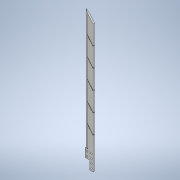
# Autodesk Inventor part: blade c 3.25
Saved by Autodesk Inventor 2021 (Build 250183000, 183)
## iProperties
Created: 2021-04-05
Part Number: blade c 3.25
Material: Generic
Document SubType Name: Modeling
Designer: newic
Density: 1 g/cm^3
Appearance: Default
Author: newic
Autodesk Inventor part; units mm, degrees
ref_plane "YZ Plane" through (0, 0, 0) normal (1, 0, 0) x (0, 1, 0)
ref_plane "XZ Plane" through (0, 0, 0) normal (0, 1, 0) x (-1, 0, 0)
ref_plane "XY Plane" through (0, 0, 0) normal (0, 0, 1) x (1, 0, 0)
sketch "Sketch1" plane through (0, 0, 0) normal (0, 0, 1) x (1, 0, 0)
  line L0 (0, 0) -> (88.9, 0)
  line L1 (88.9, 0) -> (88.9, 1168.4)
  line L2 (0, 1168.4) -> (0, 0)
  line L3 (-1378.8531, -765.1447) -> (-1378.8531, 1773.0142) construction
  line L4 (-1378.8531, 1773.0142) -> (415.5122, 1773.0142) construction
  line L5 (415.5122, 1773.0142) -> (415.5122, -765.1447) construction
  line L6 (415.5122, -765.1447) -> (-1378.8531, -765.1447) construction
  line L7 (44.45, 1168.4) -> (176.9474, 1168.4) construction
  line L8 (0, 1168.4) -> (0, 1119.7734)
  line L9 (88.9, 1168.4) -> (0, 1274.3469)
  line L10 (0, 1168.4) -> (0, 1274.3469)
  line L11 (88.9, 1168.4) -> (88.9, 1229.5585)
  line L12 (88.9, 1168.4) -> (88.9, 965.2)
  line L13 (88.9, 965.2) -> (88.9, 762)
  line L14 (88.9, 762) -> (88.9, 558.8)
  line L15 (88.9, 558.8) -> (88.9, 355.6)
  line L16 (88.9, 355.6) -> (88.9, 152.4)
  line L17 (88.9, 965.2) -> (-57.897, 1140.1458)
  line L18 (88.9, 965.2) -> (317.2756, 965.2) construction
  line L19 (88.9, 762) -> (-57.897, 936.9458)
  line L20 (88.9, 762) -> (317.2756, 762) construction
  line L21 (88.9, 558.8) -> (-71.0436, 749.4133)
  line L22 (88.9, 558.8) -> (337.728, 558.8) construction
  line L23 (88.9, 355.6) -> (-47.9591, 518.7023)
  line L24 (88.9, 355.6) -> (301.815, 355.6) construction
  line L25 (88.9, 152.4) -> (-31.1466, 295.4659)
  line L26 (88.9, 152.4) -> (275.6593, 152.4) construction
  line L27 (88.9, 152.4) -> (137.8508, 94.0627)
  line L28 (88.9, 355.6) -> (128.9332, 307.8903)
  line L29 (88.9, 558.8) -> (137.8508, 500.4627)
  line L30 (88.9, 762) -> (152.1538, 686.617)
  line L31 (-57.897, 936.9458) -> (152.1538, 686.617)
  line L32 (-71.0436, 749.4133) -> (137.8508, 500.4627)
  line L33 (-47.9591, 518.7023) -> (128.9332, 307.8903)
  line L34 (-31.1466, 295.4659) -> (137.8508, 94.0627)
  line L35 (164.9833, 874.5275) -> (-78.8863, 1165.1599)
  line L36 (90.3593, 966.4245) -> (-56.4377, 1141.3704)
  line L37 (87.4407, 963.9755) -> (-59.3563, 1138.9213)
  line L38 (157.3047, 680.4784) -> (-71.0436, 952.6133)
  line L39 (158.764, 681.7029) -> (-69.5842, 953.8378)
  line L40 (155.8454, 679.2539) -> (-72.5029, 951.3888)
  line L41 (144.9042, 492.0568) -> (-84.555, 765.5156)
  line L42 (146.3635, 493.2813) -> (-83.0956, 766.7401)
  line L43 (143.4449, 490.8323) -> (-86.0143, 764.2911)
  line L44 (137.8508, 297.2627) -> (-69.5842, 544.4742)
  line L45 (139.3101, 298.4872) -> (-68.1249, 545.6987)
  line L46 (136.3915, 296.0382) -> (-71.0436, 543.2497)
  line L47 (-41.5719, 307.8903) -> (172.2961, 53.0124)
  line L48 (-40.1126, 309.1148) -> (173.7555, 54.2369)
  line L49 (-43.0312, 306.6658) -> (170.8368, 51.7878)
  line L50 (87.4407, 963.9755) -> (94.264, 955.8438)
  dimension "d0" = 88.9
  dimension "d1" = 1168.4
  dimension "d23" = 40
  dimension "d37" = 1.905
  dimension "d38" = 1.905
  dimension "d39" = 1.905
  dimension "d40" = 1.905
  dimension "d41" = 1.905
  dimension "d42" = 1.905
  dimension "d43" = 1.905
  dimension "d44" = 1.905
  dimension "d45" = 1.905
  dimension "d46" = 1.905
  constraints: 94 end point, 11 parallel, 9 point on line, 7 horizontal, 5 equal length, 4 collinear, 3 vertical, 1 perpendicular, 2 other
  measures "d0" distance of L2.start L1.end
  measures "d1" distance of L1.end L0.end
  measures "d23" angle of L9 L11
  measures "d37" distance between parallel lines of L17 L36
  measures "d38" distance between parallel lines of L17 L37
  measures "d39" distance between parallel lines of L38 L39
  measures "d40" distance between parallel lines of L38 L40
  measures "d41" distance between parallel lines of L41 L42
  measures "d42" distance between parallel lines of L41 L43
  measures "d43" distance between parallel lines of L44 L45
  measures "d44" distance between parallel lines of L44 L46
  measures "d45" distance between parallel lines of L47 L48
  measures "d46" distance between parallel lines of L47 L49
extrude "Extrusion1" add sketch "Sketch1" along normal blind 15.875
sketch "Sketch2" plane through (0, 0, 15.875) normal (0, 0, 1) x (1, 0, 0)
  line L0 (0, 0) -> (88.9, 0)
  line L1 (88.9, 0) -> (88.9, 1168.4)
  line L2 (0, 1168.4) -> (0, 0)
  line L3 (-1378.8531, -765.1447) -> (-1378.8531, 1773.0142) construction
  line L4 (-1378.8531, 1773.0142) -> (415.5122, 1773.0142) construction
  line L5 (415.5122, 1773.0142) -> (415.5122, -765.1447) construction
  line L6 (415.5122, -765.1447) -> (-1378.8531, -765.1447) construction
  line L7 (44.45, 1168.4) -> (176.9474, 1168.4) construction
  line L8 (0, 1168.4) -> (0, 1119.7734)
  line L9 (88.9, 1168.4) -> (0, 1274.3469)
  line L10 (0, 1168.4) -> (0, 1274.3469)
  line L11 (88.9, 1168.4) -> (88.9, 1229.5585)
  line L12 (88.9, 1168.4) -> (88.9, 965.2)
  line L13 (88.9, 965.2) -> (88.9, 762)
  line L14 (88.9, 762) -> (88.9, 558.8)
  line L15 (88.9, 558.8) -> (88.9, 355.6)
  line L16 (88.9, 355.6) -> (88.9, 152.4)
  line L17 (88.9, 965.2) -> (-57.897, 1140.1458)
  line L18 (88.9, 965.2) -> (317.2756, 965.2) construction
  line L19 (88.9, 762) -> (-57.897, 936.9458)
  line L20 (88.9, 762) -> (317.2756, 762) construction
  line L21 (88.9, 558.8) -> (-71.0436, 749.4133)
  line L22 (88.9, 558.8) -> (337.728, 558.8) construction
  line L23 (88.9, 355.6) -> (-47.9591, 518.7023)
  line L24 (88.9, 355.6) -> (301.815, 355.6) construction
  line L25 (88.9, 152.4) -> (-31.1466, 295.4659)
  line L26 (88.9, 152.4) -> (275.6593, 152.4) construction
  line L27 (88.9, 152.4) -> (137.8508, 94.0627)
  line L28 (88.9, 355.6) -> (128.9332, 307.8903)
  line L29 (88.9, 558.8) -> (137.8508, 500.4627)
  line L30 (88.9, 762) -> (152.1538, 686.617)
  line L31 (-57.897, 936.9458) -> (152.1538, 686.617)
  line L32 (-71.0436, 749.4133) -> (137.8508, 500.4627)
  line L33 (-47.9591, 518.7023) -> (128.9332, 307.8903)
  line L34 (-31.1466, 295.4659) -> (137.8508, 94.0627)
  line L35 (164.9833, 874.5275) -> (-78.8863, 1165.1599)
  line L36 (90.3593, 966.4245) -> (-56.4377, 1141.3704)
  line L37 (87.4407, 963.9755) -> (-59.3563, 1138.9213)
  line L38 (157.3047, 680.4784) -> (-71.0436, 952.6133)
  line L39 (158.764, 681.7029) -> (-69.5842, 953.8378)
  line L40 (155.8454, 679.2539) -> (-72.5029, 951.3888)
  line L41 (144.9042, 492.0568) -> (-84.555, 765.5156)
  line L42 (146.3635, 493.2813) -> (-83.0956, 766.7401)
  line L43 (143.4449, 490.8323) -> (-86.0143, 764.2911)
  line L44 (137.8508, 297.2627) -> (-69.5842, 544.4742)
  line L45 (139.3101, 298.4872) -> (-68.1249, 545.6987)
  line L46 (136.3915, 296.0382) -> (-71.0436, 543.2497)
  line L47 (-41.5719, 307.8903) -> (172.2961, 53.0124)
  line L48 (-40.1126, 309.1148) -> (173.7555, 54.2369)
  line L49 (-43.0312, 306.6658) -> (170.8368, 51.7878)
  line L50 (87.4407, 963.9755) -> (94.264, 955.8438)
  point P0 (88.9, 962.2363)
  point P1 (88.9, 968.1637)
  point P2 (0, 1074.1105)
  point P3 (0, 1068.1832)
  point P4 (0, 864.9832)
  point P5 (88.9, 759.0363)
  point P6 (88.9, 764.9637)
  point P7 (0, 870.9105)
  point P8 (0, 661.7832)
  point P9 (88.9, 555.8363)
  point P10 (88.9, 561.7637)
  point P11 (0, 667.7105)
  point P12 (0, 458.5832)
  point P13 (88.9, 352.6363)
  point P14 (88.9, 358.5637)
  point P15 (0, 464.5105)
  point P16 (88.9, 155.3637)
  point P17 (0, 261.3105)
  point P18 (0, 255.3832)
  point P19 (88.9, 149.4363)
  dimension "d49" = 88.9
  dimension "d50" = 1168.4
  dimension "d51" = 40
  dimension "d52" = 1.905
  dimension "d53" = 1.905
  dimension "d54" = 1.905
  dimension "d55" = 1.905
  dimension "d56" = 1.905
  dimension "d57" = 1.905
  dimension "d58" = 1.905
  dimension "d59" = 1.905
  dimension "d60" = 1.905
  dimension "d61" = 1.905
  constraints: 94 end point, 11 parallel, 9 point on line, 7 horizontal, 5 equal length, 4 collinear, 3 vertical, 1 perpendicular, 2 other
  measures "d49" distance of L2.start L1.end
  measures "d50" distance of L1.end L0.end
  measures "d51" angle of L9 L11
  measures "d52" distance between parallel lines of L17 L36
  measures "d53" distance between parallel lines of L17 L37
  measures "d54" distance between parallel lines of L38 L39
  measures "d55" distance between parallel lines of L38 L40
  measures "d56" distance between parallel lines of L41 L42
  measures "d57" distance between parallel lines of L41 L43
  measures "d58" distance between parallel lines of L44 L45
  measures "d59" distance between parallel lines of L44 L46
  measures "d60" distance between parallel lines of L47 L48
  measures "d61" distance between parallel lines of L47 L49
extrude "Extrusion2" cut sketch "Sketch2" against normal blind 1.27 contours L2 L25 L1 L49 | L2 L48 L1 L25 | L2 L23 L1 L46 | L2 L45 L1 L23 | L2 L21 L1 L43 | L2 L42 L1 L21 | L2 L19 L1 L40 | L2 L39 L1 L19 | L2 L17 L1 L50 L37 | L2 L36 L1 L17
sketch "Sketch3" plane through (0, 0, 0) normal (0, 0, -1) x (-1, 0, 0)
  line L0 (-88.9, 149.4363) -> (0, 255.3832) projected
  line L1 (0, 261.3105) -> (-88.9, 155.3637) projected
  line L2 (0, 464.5105) -> (-88.9, 358.5637) projected
  line L3 (-88.9, 352.6363) -> (0, 458.5832) projected
  line L4 (-88.9, 555.8363) -> (0, 661.7832) projected
  line L5 (0, 667.7105) -> (-88.9, 561.7637) projected
  line L6 (-88.9, 759.0363) -> (0, 864.9832) projected
  line L7 (0, 870.9105) -> (-88.9, 764.9637) projected
  line L8 (-88.9, 962.2363) -> (0, 1068.1832) projected
  line L9 (0, 1074.1105) -> (-88.9, 968.1637) projected
  line L10 (0, 1274.3469) -> (0, 0) projected
  line L11 (-88.9, 1168.4) -> (0, 1274.3469) projected
  line L12 (-88.9, 0) -> (-88.9, 1168.4) projected
  line L13 (0, 0) -> (-88.9, 0) projected
extrude "Extrusion3" cut sketch "Sketch3" against normal blind 1.27 contours L12 L1 L10 L0 | L12 L2 L10 L3 | L12 L5 L10 L4 | L12 L7 L10 L6 | L12 L9 L10 L8
sketch "Sketch4" plane through (88.9, 968.1637, 15.875) normal (1, 0, 0) x (0, 0, -1)
  line L0 (-0.8567, 45.5077) -> (24.5433, 45.5077)
  line L1 (24.5433, 45.5077) -> (24.5433, 51.2227)
  line L2 (24.5433, 51.2227) -> (-0.8567, 51.2227)
  line L3 (-0.8567, 51.2227) -> (-0.8567, 45.5077)
  line L4 (1.27, -5.9273) -> (0, -5.9273) projected
  line L5 (0, -5.9273) -> (0, -4.4033)
  line L6 (0, 100.0196) -> (0, -97.2531) projected
  line L7 (-3.6064, -4.4033) -> (23.6569, -4.4033)
  line L8 (23.6569, -4.4033) -> (23.6569, 1.3117)
  line L9 (23.6569, 1.3117) -> (-3.6064, 1.3117)
  line L10 (-3.6064, 1.3117) -> (-3.6064, -4.4033)
  line L11 (1.27, -818.7273) -> (0, -818.7273) projected
  line L12 (0, -818.7273) -> (0, -817.2033)
  line L13 (0, -712.7804) -> (0, -968.1637) projected
  line L14 (1.27, -615.5273) -> (0, -615.5273) projected
  line L15 (0, -615.5273) -> (0, -614.0033)
  line L16 (0, -615.5273) -> (0, -509.5804) projected
  line L17 (1.27, -412.3273) -> (0, -412.3273) projected
  line L18 (0, -412.3273) -> (0, -410.8033)
  line L19 (0, -306.3804) -> (0, -503.6531) projected
  line L20 (1.27, -209.1273) -> (0, -209.1273) projected
  line L21 (0, -209.1273) -> (0, -207.6033)
  line L22 (0, -103.1804) -> (0, -300.4531) projected
  line L23 (-2.1765, -817.2033) -> (18.224, -817.2033)
  line L24 (18.224, -817.2033) -> (18.224, -811.4883)
  line L25 (18.224, -811.4883) -> (-2.1765, -811.4883)
  line L26 (-2.1765, -811.4883) -> (-2.1765, -817.2033)
  line L27 (-1.5796, -614.0033) -> (23.8204, -614.0033)
  line L28 (23.8204, -614.0033) -> (23.8204, -608.2883)
  line L29 (23.8204, -608.2883) -> (-1.5796, -608.2883)
  line L30 (-1.5796, -608.2883) -> (-1.5796, -614.0033)
  line L31 (-2.2774, -410.8033) -> (22.0155, -410.8033)
  line L32 (22.0155, -410.8033) -> (22.0155, -405.0883)
  line L33 (22.0155, -405.0883) -> (-2.2774, -405.0883)
  line L34 (-2.2774, -405.0883) -> (-2.2774, -410.8033)
  line L35 (-1.5796, -207.6033) -> (20.5708, -207.6033)
  line L36 (20.5708, -207.6033) -> (20.5708, -201.8883)
  line L37 (20.5708, -201.8883) -> (-1.5796, -201.8883)
  line L38 (-1.5796, -201.8883) -> (-1.5796, -207.6033)
  point P0 (15.875, -968.1637)
  point P1 (0, -201.8883)
  point P2 (0, -811.4883)
  point P3 (0, -608.2883)
  point P4 (0, -405.0883)
  point P5 (0, 1.3117)
  point P6 (0, -4.4033)
  dimension "d74" = 5.715
  dimension "d75" = 25.4
  dimension "d76" = 1.524
  dimension "d79" = 5.715
  dimension "d80" = 1.524
  dimension "d81" = 1.524
  dimension "d82" = 1.524
  dimension "d83" = 1.524
  dimension "d85" = 5.715
  dimension "d86" = 25.4
  dimension "d87" = 5.715
  dimension "d88" = 5.715
  dimension "d89" = 5.715
  constraints: 58 end point, 12 parallel, 6 horizontal, 6 perpendicular, 6 point on line
  measures "d74" distance of L1.end L0.end
  measures "d75" distance of L0.start L0.end
  measures "d76" distance of L4.end L5.end
  measures "d79" distance of L8.end L7.end
  measures "d80" distance of L11.end L12.end
  measures "d81" distance of L14.end L15.end
  measures "d82" distance of L17.end L18.end
  measures "d83" distance of L20.end L21.end
  measures "d85" distance of L24.end L23.end
  measures "d86" distance of L29.end L28.end
  measures "d87" distance of L28.end L27.end
  measures "d88" distance of L32.end L31.end
  measures "d89" distance of L36.end L35.end
extrude "Extrusion4" cut sketch "Sketch4" against normal blind 1.27 contours L9 L8 L7 L6 | L25 L24 L23 L13 | L16 L29 L28 L27 | L33 L32 L31 L19 | L37 L36 L35 L22
sketch "Sketch6" plane through (88.9, 766.2753, 0) normal (1, 0, 0) x (0, 0, -1)
  line L0 (-1.27, -615.315) -> (-14.605, -615.315)
  line L1 (-14.605, -615.315) -> (-14.605, -616.839)
  line L2 (-14.605, -616.839) -> (-15.875, -616.839)
  line L3 (-15.875, -766.2753) -> (-15.875, -616.839)
  line L4 (0, -766.2753) -> (-15.875, -766.2753)
  line L5 (0, -766.2753) -> (0, -616.839)
  line L6 (0, -616.839) -> (-1.27, -616.839)
  line L7 (-1.27, -616.839) -> (-1.27, -615.315)
  line L8 (-1.27, -412.115) -> (-14.605, -412.115)
  line L9 (-14.605, -412.115) -> (-14.605, -413.639)
  line L10 (-14.605, -413.639) -> (-15.875, -413.639)
  line L11 (-15.875, -609.6) -> (-15.875, -413.639)
  line L12 (-15.875, -609.6) -> (0, -609.6)
  line L13 (0, -609.6) -> (0, -413.639)
  line L14 (0, -413.639) -> (-1.27, -413.639)
  line L15 (-1.27, -413.639) -> (-1.27, -412.115)
  line L16 (0, -406.4) -> (0, -210.439)
  line L17 (-15.875, -406.4) -> (0, -406.4)
  line L18 (0, -406.4) -> (0, -210.439)
  line L19 (0, -210.439) -> (-1.27, -210.439)
  line L20 (-1.27, -210.439) -> (-1.27, -208.915)
  line L21 (-1.27, -208.915) -> (-14.605, -208.915)
  line L22 (-14.605, -208.915) -> (-14.605, -210.439)
  line L23 (-14.605, -210.439) -> (-15.875, -210.439)
  line L24 (-15.875, -406.4) -> (-15.875, -210.439)
  line L25 (-15.875, -203.2) -> (0, -203.2)
  line L26 (0, -203.2) -> (0, -7.239)
  line L27 (0, -7.239) -> (-1.27, -7.239)
  line L28 (-1.27, -7.239) -> (-1.27, -5.715)
  line L29 (-1.27, -5.715) -> (-14.605, -5.715)
  line L30 (-14.605, -5.715) -> (-14.605, -7.239)
  line L31 (-14.605, -7.239) -> (-15.875, -7.239)
  line L32 (-15.875, -203.2) -> (-15.875, -7.239)
  line L33 (-15.875, 0) -> (0, 0)
  line L34 (0, 0) -> (0, 195.961)
  line L35 (0, 195.961) -> (-1.27, 195.961)
  line L36 (-1.27, 195.961) -> (-1.27, 197.485)
  line L37 (-1.27, 197.485) -> (-14.605, 197.485)
  line L38 (-14.605, 197.485) -> (-14.605, 195.961)
  line L39 (-14.605, 195.961) -> (-15.875, 195.961)
  line L40 (-15.875, 0) -> (-15.875, 195.961)
  line L41 (-15.875, 203.2) -> (0, 203.2)
  line L42 (0, 203.2) -> (0, 402.1247)
  line L43 (0, 402.1247) -> (-15.875, 402.1247)
  line L44 (-15.875, 203.2) -> (-15.875, 402.1247)
  line L45 (0, 402.1247) -> (0, 508.0715)
  line L46 (0, 508.0715) -> (-15.875, 508.0715)
  line L47 (-15.875, 402.1247) -> (-15.875, 508.0715)
  line L48 (0, 402.1247) -> (-15.875, 402.1247)
  line L49 (-15.875, 195.961) -> (-15.875, 301.9079)
  line L50 (0, 195.961) -> (-1.27, 195.961)
  line L51 (-15.875, 197.485) -> (0, 197.485)
  line L52 (0, 197.485) -> (0, 195.961)
  line L53 (0, 195.961) -> (-15.875, 195.961)
  line L54 (-15.875, 195.961) -> (-15.875, 197.485)
  line L55 (-15.875, 98.7079) -> (-15.875, -98.5648)
  line L56 (0, -7.239) -> (-1.27, -7.239)
  line L57 (-15.875, -5.715) -> (0, -5.715)
  line L58 (0, -5.715) -> (0, -7.239)
  line L59 (0, -7.239) -> (-15.875, -7.239)
  line L60 (-15.875, -7.239) -> (-15.875, -5.715)
  line L61 (-15.875, -104.4921) -> (-15.875, -301.7648)
  line L62 (0, -104.4921) -> (0, -210.439)
  line L63 (-15.875, -208.915) -> (0, -208.915)
  line L64 (0, -208.915) -> (0, -210.439)
  line L65 (0, -210.439) -> (-15.875, -210.439)
  line L66 (-15.875, -210.439) -> (-15.875, -208.915)
  line L67 (-15.875, -413.639) -> (-15.875, -307.6921)
  line L68 (0, -307.6921) -> (0, -413.639)
  line L69 (-15.875, -412.115) -> (0, -412.115)
  line L70 (0, -412.115) -> (0, -413.639)
  line L71 (0, -413.639) -> (-15.875, -413.639)
  line L72 (-15.875, -413.639) -> (-15.875, -412.115)
  line L73 (-15.875, -616.839) -> (-15.875, -510.8921)
  line L74 (0, -510.8921) -> (0, -616.839)
  line L75 (-15.875, -615.315) -> (0, -615.315)
  line L76 (0, -615.315) -> (0, -616.839)
  line L77 (0, -616.839) -> (-15.875, -616.839)
  line L78 (-15.875, -616.839) -> (-15.875, -615.315)
extrude "Extrusion5" add sketch "Sketch6" against normal blind 1.27 contours L7 L77 L1 L0 | L75 L74 L6 L7 | L1 L2 L73 L75 | L14 L15 L69 L68 | L67 L69 L9 L10 | L71 L9 L8 L15 | L19 L20 L63 L62 | L65 L22 L21 L20 | L61 L63 L22 L23 | L27 L28 L57 L58 | L59 L30 L29 L28 | L55 L57 L30 L31 | L35 L36 L51 L52 | L49 L51 L38 L39 | L53 L38 L37 L36
sketch "Sketch8" plane through (0, 0, 15.875) normal (0, 0, 1) x (1, 0, 0)
  line L0 (0, -7.1275) -> (6.35, -7.1275)
  line L1 (6.35, -7.1275) -> (6.35, 1442.9398)
  line L2 (6.35, 1442.9398) -> (0, 1442.9398)
  line L3 (0, 1442.9398) -> (0, -7.1275)
  point P0 (0, 0)
  dimension "d94" = 6.35
  constraints: 8 end point, 2 parallel, 1 horizontal, 1 perpendicular
  measures "d94" distance of L2.end L1.end
extrude "Extrusion6" cut sketch "Sketch8" against normal through all
sketch "Sketch12" plane through (88.9, 0, 0) normal (0, -1, 0) x (1, 0, 0)
  line L0 (-82.55, 15.875) -> (-82.55, 14.605) projected
  line L1 (-82.55, 15.875) -> (-57.15, 15.875)
  line L2 (-82.55, 15.875) -> (-1.1006, 15.875) projected
  line L3 (-57.15, 15.875) -> (-82.55, 7.9375)
  line L4 (-82.55, 15.875) -> (-82.55, 0) projected
  line L5 (-82.55, 0) -> (-1.27, 0) projected
  line L6 (-82.55, 15.875) -> (-82.55, 0) projected
  line L7 (-82.55, 0) -> (0, 0) projected
  line L8 (0, 0) -> (0, 15.875) projected
  line L9 (-82.55, 15.875) -> (0, 15.875) projected
  line L10 (-57.15, 0) -> (-82.55, 7.9375)
  point P0 (-88.9, 0)
  dimension "d104" = 25.4
  constraints: 6 end point, 2 point on line, 1 midpoint
  measures "d104" distance of L0.start L1.end
extrude "Extrusion8" cut sketch "Sketch12" against normal through all contours L1 L3 L4 L0 | L10 L5 L4
sketch "Sketch13" plane through (88.9, 0, 0) normal (0, -1, 0) x (1, 0, 0)
  line L0 (0, 0) -> (0, 15.875) projected
  line L1 (0, 0) -> (-82.55, 0)
  line L2 (-82.55, 0) -> (-82.55, 15.875)
  line L3 (-82.55, 15.875) -> (0, 15.875)
  line L4 (0, 15.875) -> (0, 0)
  point P0 (-88.9, 0)
  constraints: 8 end point, 2 parallel, 1 horizontal, 1 perpendicular
extrude "Extrusion9" add sketch "Sketch13" along normal blind 184.15
sketch "Sketch14" plane through (0, 0, 15.875) normal (0, 0, 1) x (1, 0, 0)
  line L0 (6.35, 0) -> (6.35, -184.15) projected
  line L1 (6.35, 0) -> (6.35, -91.44)
  line L2 (6.35, -91.44) -> (52.07, -91.44)
  line L3 (52.07, -91.44) -> (52.07, -182.88)
  line L4 (52.07, -182.88) -> (88.9, -182.88)
  line L5 (88.9, 150.9603) -> (88.9, -184.15) projected
  line L6 (31.75, 217.5451) -> (31.75, 0) projected
  line L7 (31.75, 0) -> (6.35, 0) projected
  line L8 (6.35, 0) -> (6.35, -184.15) projected
  line L9 (88.9, -184.15) -> (6.35, -184.15) projected
  line L10 (88.9, 150.9603) -> (88.9, -184.15) projected
  line L11 (88.9, 150.9603) -> (87.63, 150.9603) projected
  line L12 (87.63, 150.9499) -> (87.63, 150.9603) projected
  line L13 (87.63, 150.9499) -> (31.75, 217.5451) projected
  point P0 (0, 0)
  dimension "d109" = 91.44
  dimension "d112" = 45.72
  dimension "d113" = 91.44
  constraints: 8 end point, 2 perpendicular, 2 point on line, 1 horizontal
  measures "d109" distance of L0.start L1.end
  measures "d112" distance of L1.end L2.end
  measures "d113" distance of L2.end L3.end
extrude "Extrusion10" cut sketch "Sketch14" against normal blind 184.15 contours L2 L3 L4 L5 L9 L0
sketch "Sketch17" plane through (0, 0, 15.875) normal (0, 0, 1) x (1, 0, 0)
  line L0 (6.35, 0) -> (6.35, -91.44) projected
  line L1 (47.625, -45.72) -> (6.35, -45.72)
  line L2 (6.35, -45.72) -> (6.35, 0)
  line L3 (6.35, 0) -> (47.625, 0)
  line L4 (47.625, 0) -> (47.625, -45.72)
  line L5 (88.9, 150.9603) -> (88.9, -182.88) projected
  line L6 (47.625, -45.72) -> (88.9, -45.72)
  line L7 (88.9, -45.72) -> (88.9, 0)
  line L8 (88.9, 0) -> (47.625, 0)
  line L9 (47.625, 0) -> (47.625, -45.72)
  line L10 (47.625, -45.72) -> (88.9, -45.72)
  line L11 (88.9, -45.72) -> (88.9, -91.44)
  line L12 (88.9, -91.44) -> (47.625, -91.44)
  line L13 (47.625, -91.44) -> (47.625, -45.72)
  line L14 (6.35, -91.44) -> (52.07, -91.44) projected
  line L15 (47.625, -45.72) -> (6.35, -45.72)
  line L16 (6.35, -45.72) -> (6.35, -91.44)
  line L17 (6.35, -91.44) -> (47.625, -91.44)
  line L18 (47.625, -91.44) -> (47.625, -45.72)
  line L19 (52.07, -182.88) -> (88.9, -182.88)
  line L20 (88.9, -182.88) -> (88.9, -137.16)
  line L21 (88.9, -137.16) -> (52.07, -137.16)
  line L22 (52.07, -137.16) -> (52.07, -182.88)
  line L23 (52.07, -137.16) -> (88.9, -137.16)
  line L24 (88.9, -137.16) -> (88.9, -91.44)
  line L25 (88.9, -91.44) -> (52.07, -91.44)
  line L26 (52.07, -91.44) -> (52.07, -137.16)
  circle A0 centre (26.9875, -22.86) radius 8.255
  circle A1 centre (70.485, -22.86) radius 8.255
  circle A2 centre (70.485, -68.58) radius 8.255
  circle A3 centre (26.9875, -68.58) radius 8.255
  circle A4 centre (70.485, -114.3) radius 8.255
  circle A5 centre (70.485, -160.02) radius 8.255
  point P0 (70.485, -137.16)
  dimension "d120" = 16.51
  dimension "d121" = 16.51
  dimension "d122" = 16.51
  dimension "d123" = 16.51
  dimension "d124" = 16.51
  dimension "d125" = 16.51
  constraints: 48 end point, 12 parallel, 6 centre point, 6 coincident, 6 horizontal, 6 perpendicular, 4 point on line
  measures "d120" diameter of A0
  measures "d121" diameter of A1
  measures "d122" diameter of A4
  measures "d123" diameter of A5
  measures "d124" diameter of A2
  measures "d125" diameter of A3
extrude "Extrusion11" cut sketch "Sketch17" against normal blind 25.4 contours A0 | A1 | A2 | A3 | A4 | A5
body "Solid1"
